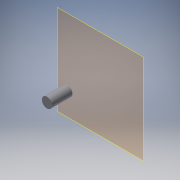
# Autodesk Inventor part: peg(working)
Saved by Autodesk Inventor 2017 (Build 210142000, 142)
## iProperties
Created: 2017-01-16
Part Number: peg(working)
Material: Generic
Document SubType Name: Modeling
Designer: kingb
Density: 1 g/cm^3
Appearance: Default
Author: kingb
Autodesk Inventor part; units mm, degrees
ref_plane "YZ Plane" through (0, 0, 0) normal (1, 0, 0) x (0, 1, 0)
ref_plane "XZ Plane" through (0, 0, 0) normal (0, 1, 0) x (-1, 0, 0)
ref_plane "Work Plane1" through (12.6214, -14.8597, 0) normal (0, 0, 1) x (1, 0, 0)
sketch "Sketch1" plane through (12.6214, -14.8597, 0) normal (0, 0, 1) x (1, 0, 0)
  circle A0 centre (-122.428, -92.9546) radius 19.05
  point P0 (-12.6214, 14.8597)
  dimension "d0" = 38.1
  constraints: 1 centre point
  measures "d0" diameter of A0
extrude "Extrusion1" add sketch "Sketch1" along normal blind 76.2
body "Solid1"
